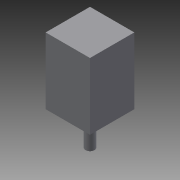
# Autodesk Inventor part: NEMA8
Saved by Autodesk Inventor 2014 SP2 (Build 180246200, 246)
## iProperties
Created: 2015-11-29
Part Number: NEMA8
Material: Generic
Document SubType Name: Modeling
Designer: schrluka
Density: 1 g/cm^3
Appearance: Default
Author: schrluka
Autodesk Inventor part; units mm, degrees
ref_plane "YZ Plane" through (0, 0, 0) normal (1, 0, 0) x (0, 1, 0)
ref_plane "XZ Plane" through (0, 0, 0) normal (0, 1, 0) x (-1, 0, 0)
ref_plane "XY Plane" through (0, 0, 0) normal (0, 0, 1) x (1, 0, 0)
sketch "Sketch1" plane through (0, 0, 0) normal (0, 0, 1) x (1, 0, 0)
  line L0 (-10, -10) -> (10, -10)
  line L1 (10, -10) -> (10, 10)
  line L2 (10, 10) -> (-10, 10)
  line L3 (-10, 10) -> (-10, -10)
  line L4 (-10, -10) -> (10, 10) construction
  line L5 (10, -10) -> (-10, 10) construction
  point P0 (0, 0)
  dimension "d0" = 20
  dimension "d1" = 20
  constraints: 12 end point, 2 midpoint, 2 parallel, 1 horizontal, 1 perpendicular
  measures "d0" distance of L2.end L1.end
  measures "d1" distance of L1.end L0.end
extrude "Extrusion1" add sketch "Sketch1" along normal blind 30
sketch "Sketch2" plane through (0, 0, 0) normal (0, 0, -1) x (-1, 0, 0)
  point P0 (0, 0)
  point P1 (-8, 8)
  point P2 (8, 8)
  point P3 (8, -8)
  point P4 (-8, -8)
  dimension "d4" = 8
  dimension "d5" = 8
  dimension "d6" = 8
  dimension "d7" = 8
  dimension "d8" = 8
  dimension "d9" = 8
  dimension "d10" = 8
  dimension "d11" = 8
  measures "d4" horizontal distance of point (0, 0) point (-8, 8)
  measures "d5" horizontal distance of point (8, 8) point (0, 0)
  measures "d6" horizontal distance of point (8, -8) point (0, 0)
  measures "d7" horizontal distance of point (0, 0) point (-8, -8)
  measures "d8" horizontal distance of point (-8, -8) point (0, 0)
  measures "d9" horizontal distance of point (8, -8) point (0, 0)
  measures "d10" horizontal distance of point (8, 8) point (0, 0)
  measures "d11" horizontal distance of point (0, 0) point (-8, 8)
hole "Hole1" at (8, 8, 0) at (-8, 8, 0) at (-8, -8, 0) at (8, -8, 0) direction (0, 0, 1) diameter 2 depth 3.5 tip angle 118
sketch "Sketch3" plane through (0, 0, 0) normal (0, 0, -1) x (-1, 0, 0)
  circle A0 centre (0, 0) radius 7.5
  dimension "d19" = 15
  constraints: 1 centre point, 1 coincident
  measures "d19" diameter of A0
extrude "Extrusion2" add sketch "Sketch3" along normal blind 1.5
sketch "Sketch4" plane through (0, 0, -1.5) normal (0, 0, -1) x (-1, 0, 0)
  circle A0 centre (0, 0) radius 7.5 projected
  circle A1 centre (0, 0) radius 2
  dimension "d22" = 4
  constraints: 1 centre point, 1 coincident
  measures "d22" diameter of A1
extrude "Extrusion3" add sketch "Sketch4" along normal blind 13.5 contours A1
body "Solid1"
